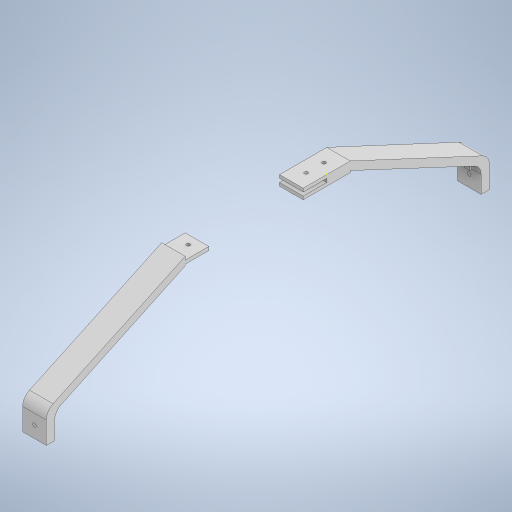
# Autodesk Inventor part: trem de pouso
Saved by Autodesk Inventor 2024.3 (Build 283343000, 343)
## iProperties
Created: 2024-08-27
Part Number: trem de pouso
Material: Genérico
Document SubType Name: Modeling
Designer: Sabio
Density: 1 g/cm^3
Appearance: Padrão
Author: Sabio
Autodesk Inventor part; units mm, degrees
ref_plane "YZ Plane" through (0, 0, 0) normal (1, 0, 0) x (0, 1, 0)
ref_plane "XZ Plane" through (0, 0, 0) normal (0, 1, 0) x (-1, 0, 0)
sketch "Esboço1" plane through (0, 0, 0) normal (1, 0, 0) x (0, 1, 0)
  line L0 (-0.3925, -0.0182) -> (-0.3925, -20.0182)
  line L1 (-0.3925, -20.0182) -> (-55.3328, -137.8382)
  line L2 (-0.3925, -20.0182) -> (-0.3925, -117.6672) construction
  line L3 (-55.3328, -137.8382) -> (-80.3328, -137.8382)
  line L4 (-80.3328, -137.8382) -> (-80.3328, -130.8382)
  line L5 (-80.3328, -130.8382) -> (-59.2983, -130.8382)
  line L6 (-59.2983, -130.8382) -> (-7.3925, -20.0182)
  line L7 (-7.3925, -20.0182) -> (-7.3925, -0.0182)
  line L8 (-0.3925, -0.0182) -> (-0.3925, 19.9818)
  line L9 (-0.3925, 19.9818) -> (-55.3328, 137.8018)
  line L10 (-55.3328, 137.8018) -> (-80.3328, 137.8018)
  line L11 (-80.3328, 137.8018) -> (-80.3328, 130.8018)
  line L12 (-80.3328, 130.8018) -> (-59.2983, 130.8018)
  line L13 (-59.2983, 130.8018) -> (-7.3925, 19.9818)
  line L14 (-7.3925, 19.9818) -> (-7.3925, -0.0182)
  point P0 (0, 0)
  point P1 (-7.3925, -10.0182)
  dimension "d0" = 20
  dimension "d2" = 130
  dimension "d3" = 25
  dimension "d4" = 25
  dimension "d5" = 7
  dimension "d6" = 0.097
  dimension "d7" = 7
  dimension "d8" = 25
  constraints: 30 end point, 3 vertical, 1 horizontal, 1 midpoint, 1 parallel, 1 perpendicular
  measures "d0" distance of L0.start L0.end
  measures "d2" distance of L0.end L1.end
  measures "d3" angle of L1 L2
  measures "d4" distance of L1.end L3.end
  measures "d5" distance of L3.end L4.end
  measures "d6" angle of L1 L6
  measures "d7" distance from line of point (-7.392, -10.018) L0
  measures "d8" distance of L10.end L9.end
extrude "Extrusão1" add sketch "Esboço1" along normal blind 20
sketch "Esboço2" plane through (0, -0.3925, 19.9818) normal (0, 1, 0) x (1, 0, 0)
  circle A0 centre (10, 12.5) radius 1.75
  circle A1 centre (10, 27.5) radius 1.75
  line L0 (0, 40) -> (0, 0) projected
  line L1 (0, 0) -> (20, 0) projected
  line L2 (0, 40) -> (20, 40) projected
  point P0 (0, 19.9818)
  point P1 (10, 0)
  point P2 (10, 40)
  dimension "d11" = 15
  dimension "d12" = 3.5
  dimension "d13" = 3.5
  dimension "d14" = 10
  dimension "d15" = 10
  dimension "d16" = 12.5
  dimension "d17" = 12.5
  constraints: 2 centre point, 2 midpoint
  measures "d11" distance of A1.centre A0.centre
  measures "d12" diameter of A0
  measures "d13" diameter of A1
  measures "d14" distance from line of L0 A0.centre
  measures "d15" distance from line of L0 A1.centre
  measures "d16" distance of point (10, 0) A0.centre
  measures "d17" distance of point (10, 40) A1.centre
hole "Furo1" at (10, -0.3925, 7.4818) at (10, -0.3925, -7.5182) direction (0, -1, 0) diameter 3 end through all
sketch "Esboço3" plane through (0, -80.3328, 137.8018) normal (0, 0, 1) x (1, 0, 0)
  circle A0 centre (10, 10) radius 1.75
  line L0 (0, 25) -> (0, 0) projected
  line L1 (20, 25) -> (20, 0) projected
  line L2 (0, 0) -> (20, 0) projected
  point P0 (0, 80.3328)
  dimension "d27" = 3.5
  dimension "d28" = 10
  dimension "d29" = 10
  dimension "d30" = 10
  constraints: 1 centre point
  measures "d27" diameter of A0
  measures "d28" distance from line of L0 A0.centre
  measures "d29" distance from line of L1 A0.centre
  measures "d30" distance from line of L2 A0.centre
hole "Furo2" at (10, -70.3328, 137.8018) direction (0, 0, -1) diameter 3 end through all
sketch "Esboço5" plane through (0, -59.2983, -130.8382) normal (0, -0.9055877, 0.4241591) x (1, 0, 0)
  line L0 (0, 122.3736) -> (20, 122.3736) projected
  line L1 (0, 0) -> (20, 0) projected
  line L2 (7.8224, 122.3736) -> (11.9968, 122.3736)
  line L3 (11.9968, 122.3736) -> (11.9968, 0)
  line L4 (11.9968, 0) -> (7.8224, 0)
  line L5 (7.8224, 0) -> (7.8224, 122.3736)
  point P0 (0, 143.6374)
  constraints: 8 end point, 2 parallel, 2 point on line, 1 horizontal, 1 perpendicular
extrude "Extrusão2" add sketch "Esboço5" along normal blind 1.5
sketch "Esboço7" plane through (0, -80.3328, -130.8382) normal (0, 0, 1) x (1, 0, 0)
  line L0 (7.8224, 21.0345) -> (7.8224, 19.6761) projected
  line L1 (7.8224, 21.0345) -> (7.8224, 14.1441)
  line L2 (11.9968, 21.0345) -> (11.9968, 19.6761) projected
  line L3 (11.9968, 21.0345) -> (11.9968, 14.1441)
  line L4 (11.9968, 14.1441) -> (7.8224, 14.1441)
  line L5 (0, 21.0345) -> (7.8224, 21.0345) projected
  line L6 (7.8224, 21.0345) -> (11.9968, 21.0345)
  point P0 (0, 80.3328)
  constraints: 8 end point, 2 collinear, 2 perpendicular
extrude "Extrusão4" add sketch "Esboço7" along normal blind 1.5
sketch "Esboço8" plane through (0, -7.3925, 19.9818) normal (0, -0.9055877, -0.4241591) x (1, 0, 0)
  line L0 (0, 0) -> (20, 0) projected
  line L1 (0, 122.3736) -> (20, 122.3736) projected
  line L2 (11.997, 0) -> (8.003, 0)
  line L3 (8.003, 0) -> (8.003, 122.3736)
  line L4 (8.003, 122.3736) -> (11.997, 122.3736)
  line L5 (11.997, 122.3736) -> (11.997, 0)
  line L6 (20, 122.3736) -> (20, 0) projected
  line L7 (0, 122.3736) -> (0, 0) projected
  point P0 (0, -21.2309)
  point P1 (11.997, 61.1868)
  dimension "d58" = 8.003
  dimension "d59" = 8.003
  constraints: 8 end point, 2 parallel, 2 point on line, 1 horizontal, 1 midpoint, 1 perpendicular
  measures "d58" distance from line of point (11.997, 61.187) L6
  measures "d59" distance between parallel lines of L7 L3
extrude "Extrusão5" add sketch "Esboço8" along normal blind 1.5 contours L3 L1 L5 L0
sketch "Esboço11" plane through (0, -80.3328, 130.8018) normal (0, 0, -1) x (-1, 0, 0)
  line L0 (0, 21.0345) -> (-8.003, 21.0345) projected
  line L1 (-8.003, 21.0345) -> (-8.003, 15.1045)
  line L2 (-11.997, 21.0345) -> (-20, 21.0345) projected
  line L3 (-11.997, 21.0345) -> (-11.997, 15.1045)
  line L4 (-11.997, 15.1045) -> (-8.003, 15.1045)
  line L5 (-8.003, 21.0345) -> (-11.997, 21.0345) projected
  line L6 (-11.997, 21.0345) -> (-8.003, 21.0345)
  point P0 (0, 80.3328)
  point P1 (-10, 15.1045)
  dimension "d64" = 5.93
  constraints: 8 end point, 2 vertical, 1 horizontal, 1 midpoint, 1 perpendicular
  measures "d64" distance from line of point (-10, 15.104) L5
extrude "Extrusão7" add sketch "Esboço11" along normal blind 1.5
fillet "Arredondamento12" radius 2 1 edges at (10, -60.2522, 129.3018)
fillet "Arredondamento13" radius 2 1 edges at (9.9096, -60.2522, -129.3382)
sketch "Esboço12" plane through (0, -7.3925, -20.0182) normal (0, -1, 0) x (1, 0, 0)
  line L0 (0, 40) -> (20, 40) projected
  line L1 (0, 0) -> (1.5, 0)
  line L2 (1.5, 1.5) -> (1.5, 38.5)
  line L3 (1.5, 40) -> (0, 40)
  line L4 (0, 40) -> (0, 0)
  line L5 (0, 0) -> (20, 0) projected
  line L6 (20, 0) -> (18.5, 0)
  line L7 (18.5, 1.5) -> (18.5, 38.5)
  line L8 (18.5, 40) -> (20, 40)
  line L9 (20, 40) -> (20, 0)
  line L10 (1.5, 0) -> (18.5, 0)
  line L11 (18.5, 1.5) -> (1.5, 1.5)
  line L12 (1.5, 40) -> (18.5, 40)
  line L13 (18.5, 38.5) -> (1.5, 38.5)
  point P0 (0, 20.0182)
  dimension "d70" = 1.5
  dimension "d71" = 1.5
  dimension "d72" = 1.5
  dimension "d73" = 1.5
  constraints: 24 end point, 6 parallel, 4 horizontal, 2 perpendicular, 2 point on line
  measures "d70" distance between parallel lines of L4 L2
  measures "d71" distance between parallel lines of L9 L7
  measures "d72" distance between parallel lines of L11 L10
  measures "d73" distance between parallel lines of L0 L13
extrude "Extrusão8" add sketch "Esboço12" along normal blind 1.5
ref_plane "Plano de trabalho1" through (424, 0, 0) normal (1, 0, 0) x (0, 0, -1)
fillet "Arredondamento17" radius 10 6 edges at (10, -55.3328, 137.8018) (15.9985, -59.2983, 130.8018) (4.0015, -59.2983, 130.8018) (10, -55.3328, -137.8382) (15.9984, -59.2983, -130.8382) (3.9112, -59.2983, -130.8382)
sketch "Esboço28" plane through (20, 0, 0) normal (1, 0, 0) x (0, 0, -1)
  point P0 (0, 0)
sketch "Esboço29" plane through (20, 0, 0) normal (1, 0, 0) x (0, 0, -1)
  line L0 (0.0182, -3.146) -> (0.0182, -6.1389)
  line L1 (-19.9818, -3.146) -> (0.0182, -3.146)
  line L2 (0.0182, -6.1389) -> (-19.9818, -6.1389)
  line L3 (-19.9818, -9.5301) -> (-19.9818, -6.1389)
  line L4 (-19.9818, -3.146) -> (-19.9818, -0.3925)
  line L5 (-19.9818, -0.3925) -> (-19.9818, 0)
  point P0 (0, 0)
  constraints: 12 end point, 2 vertical, 1 horizontal, 1 parallel
split body "Dividir1" sketch "Esboço29" result two bodies curves L3 L2 L0 L1 L4 L5 first body at (13.3333, -18.2616, 57.1192)
move or copy body "Deslocar corpo1" bodies to move or copy 2 copy no translate (0, 0, 100)
